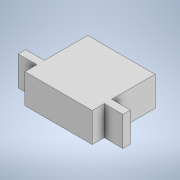
# Autodesk Inventor part: EMAXES9251
Saved by Autodesk Inventor 2021 (Build 250183000, 183)
## iProperties
Created: 2020-11-13
Part Number: EMAXES9251
Material: Generic
Document SubType Name: Modeling
Designer: Paco
Density: 1 g/cm^3
Appearance: Default
Author: Paco
Autodesk Inventor part; units mm, degrees
ref_plane "YZ Plane" through (0, 0, 0) normal (1, 0, 0) x (0, 1, 0)
ref_plane "XZ Plane" through (0, 0, 0) normal (0, 1, 0) x (-1, 0, 0)
ref_plane "XY Plane" through (0, 0, 0) normal (0, 0, 1) x (1, 0, 0)
sketch "Sketch1" plane through (0, 0, 0) normal (0, 1, 0) x (-1, 0, 0)
  line L0 (-19.3459, 17.7433) -> (-1.3259, 17.7433)
  line L1 (-1.3259, 0.9433) -> (-19.3459, 0.9433)
  line L2 (-19.3459, 14.5433) -> (-24.3459, 14.5433)
  line L3 (-24.3459, 14.5433) -> (-24.3459, 12.5433)
  line L4 (-24.3459, 12.5433) -> (-19.3459, 12.5433)
  line L5 (-19.3459, 17.7433) -> (-19.3459, 14.5433)
  line L6 (-19.3459, 12.5433) -> (-19.3459, 0.9433)
  line L7 (-1.3259, 17.7433) -> (-1.3259, 14.5433)
  line L8 (-1.3259, 14.5433) -> (3.6741, 14.5433)
  line L9 (3.6741, 14.5433) -> (3.6741, 12.5433)
  line L10 (3.6741, 12.5433) -> (-1.3259, 12.5433)
  line L11 (-1.3259, 12.5433) -> (-1.3259, 0.9433)
  point P0 (0, 0)
  point P1 (-11, -1)
  dimension "d0" = 18.02
  dimension "d1" = 16.8
  dimension "d2" = 2
  dimension "d3" = 5
  dimension "d4" = 3.2
  constraints: 24 end point, 2 horizontal, 2 parallel, 1 collinear, 1 perpendicular, 1 vertical
  measures "d0" distance of L0.start L0.end
  measures "d1" distance between parallel lines of L1 L0
  measures "d2" distance of L2.end L3.end
  measures "d3" distance of L3.end L4.end
  measures "d4" distance of L0.start L2.start
extrude "Extrusion1" add sketch "Sketch1" along normal blind 7.91
body "Solid1"
